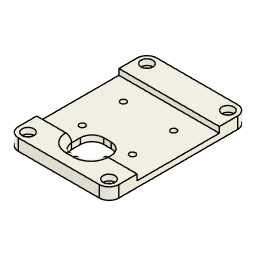
LINK-SHELF-to-B_ADPTOR (Autodesk Fusion 360 design; units mm, degrees)
Autodesk Fusion 360 part; units mm, degrees
sketch "Sketch1" plane through (0, 0, 9.3444) normal (0, 0, 1) x (1, 0, 0)
  circle A0 centre (-20.83, 96.1191) radius 1.5
  circle A1 centre (-20.83, 157.2691) radius 1.5
  circle A2 centre (20.83, 96.1191) radius 1.5
  circle A3 centre (20.83, 157.2691) radius 1.5
  line L0 (-15, 155.8968) -> (-15, 157.1191)
  line L1 (-15, 157.1191) -> (15, 157.1191)
  line L2 (15, 157.1191) -> (15, 155.8968)
  line L3 (15, 155.8968) -> (-15, 155.8968)
  arc A4 (25.83, 157.2691) -> (20.83, 162.2691) centre (20.83, 157.2691) ccw
  line L4 (20.83, 162.2691) -> (-20.83, 162.2691)
  arc A5 (-20.83, 162.2691) -> (-25.83, 157.2691) centre (-20.83, 157.2691) ccw
  line L5 (-25.83, 157.2691) -> (-25.83, 96.1191)
  arc A6 (-25.83, 96.1191) -> (-20.83, 91.1191) centre (-20.83, 96.1191) ccw
  line L6 (-20.83, 91.1191) -> (20.83, 91.1191)
  arc A7 (20.83, 91.1191) -> (25.83, 96.1191) centre (20.83, 96.1191) ccw
  line L7 (25.83, 96.1191) -> (25.83, 157.2691)
  line L8 (11.75, 110.7057) -> (11.75, 99.7057)
  line L9 (11.75, 99.7057) -> (0.75, 99.7057)
  line L10 (0.75, 99.7057) -> (0.75, 110.7057)
  line L11 (-0.75, 110.7057) -> (-0.75, 99.7057)
  line L12 (-0.75, 99.7057) -> (-11.75, 99.7057)
  line L13 (-11.75, 99.7057) -> (-11.75, 110.7057)
  line L14 (8.8, 110.7057) -> (11.75, 110.7057)
  line L15 (0.75, 110.7057) -> (3.7, 110.7057)
  line L16 (-3.7, 110.7057) -> (-0.75, 110.7057)
  line L17 (-11.75, 110.7057) -> (-8.8, 110.7057)
  line L18 (3.7, 110.7057) -> (3.7, 139.7691)
  line L19 (3.7, 139.7691) -> (8.8, 139.7691)
  line L20 (8.8, 139.7691) -> (8.8, 110.7057)
  line L21 (-8.8, 110.7057) -> (-8.8, 139.7691)
  line L22 (-8.8, 139.7691) -> (-3.7, 139.7691)
  line L23 (-3.7, 139.7691) -> (-3.7, 110.7057)
extrude "Extrude1" add sketch "Sketch1" along normal blind 3 contours L0 L1 L2 L3 | A4 L4 A5 L5 A6 L6 A7 L7 | L8 L9 L10 L14 L15 L18 L19 L20 | L11 L12 L13 L16 L17 L21 L22 L23
sketch "Sketch2" plane through (0, 0, 12.3444) normal (0, 0, 1) x (-1, 0, 0)
  circle A0 centre (20.83, -157.2691) radius 1.5
  circle A1 centre (20.83, -96.1191) radius 1.5
  circle A2 centre (-20.83, -157.2691) radius 1.5
  circle A3 centre (-20.83, -96.1191) radius 1.5
  line L0 (-25.83, -96.1191) -> (-25.83, -157.2691)
  arc A4 (-25.83, -157.2691) -> (-20.83, -162.2691) centre (-20.83, -157.2691) ccw
  line L1 (-20.83, -162.2691) -> (20.83, -162.2691)
  arc A5 (20.83, -162.2691) -> (25.83, -157.2691) centre (20.83, -157.2691) ccw
  line L2 (25.83, -157.2691) -> (25.83, -96.1191)
  arc A6 (25.83, -96.1191) -> (20.83, -91.1191) centre (20.83, -96.1191) ccw
  line L3 (20.83, -91.1191) -> (-20.83, -91.1191)
  arc A7 (-20.83, -91.1191) -> (-25.83, -96.1191) centre (-20.83, -96.1191) ccw
  line L4 (-25.83, -126.6941) -> (25.83, -126.6941) construction
  line L5 (0, -126.6941) -> (0, -105.5441) construction
  line L6 (0, -126.6941) -> (0, -147.8441) construction
  line L7 (-25.83, -105.5441) -> (25.83, -105.5441)
  line L8 (25.83, -105.5441) -> (25.83, -147.8441)
  line L9 (25.83, -147.8441) -> (-25.83, -147.8441)
  line L10 (-25.83, -147.8441) -> (-25.83, -105.5441)
  dimension "d41" = 21.15
  dimension "d42" = 21.15
  constraint midpoint L0 L4.start
  constraint midpoint L2 L4.end
  constraint midpoint L4 L5.start
  constraint perpendicular L4 L5
  constraint perpendicular L4 L6
  constraint horizontal L7
  constraint vertical L8
  constraint horizontal L9
  constraint vertical L10
  constraint coincident L2 L8.end
  constraint coincident L0 L7.start
  measures "d41" distance of L5.start L5.end
  measures "d42" distance of L5.start L6.end
extrude "Extrude2" add sketch "Sketch2" along normal blind 3 contours L0 L2 A6 L3 A7 L7 | L0 A4 L1 A5 L2 L9
sketch "Sketch3" plane through (0, 0, 15.3444) normal (0, 0, 1) x (-1, 0, 0)
  circle A0 centre (-20.83, -157.2691) radius 1.5
  circle A1 centre (20.83, -157.2691) radius 1.5
  line L0 (25.83, -147.8441) -> (-25.83, -147.8441)
  line L1 (-25.83, -147.8441) -> (-25.83, -157.2691)
  arc A2 (-25.83, -157.2691) -> (-20.83, -162.2691) centre (-20.83, -157.2691) ccw
  line L2 (-20.83, -162.2691) -> (20.83, -162.2691)
  arc A3 (20.83, -162.2691) -> (25.83, -157.2691) centre (20.83, -157.2691) ccw
  line L3 (25.83, -157.2691) -> (25.83, -147.8441)
  circle A4 centre (-20.83, -96.1191) radius 1.5
  circle A5 centre (20.83, -96.1191) radius 1.5
  line L4 (-25.83, -105.5441) -> (25.83, -105.5441)
  line L5 (25.83, -105.5441) -> (25.83, -96.1191)
  arc A6 (25.83, -96.1191) -> (20.83, -91.1191) centre (20.83, -96.1191) ccw
  line L6 (20.83, -91.1191) -> (-20.83, -91.1191)
  arc A7 (-20.83, -91.1191) -> (-25.83, -96.1191) centre (-20.83, -96.1191) ccw
  line L7 (-25.83, -96.1191) -> (-25.83, -105.5441)
  circle A8 centre (-20.83, -157.2691) radius 3.05
  circle A9 centre (20.83, -157.2691) radius 3.05
  circle A10 centre (-20.83, -96.1191) radius 3.05
  circle A11 centre (20.83, -96.1191) radius 3.05
  dimension "d45" = 6.1
  dimension "d46" = 6.1
  dimension "d47" = 6.1
  dimension "d48" = 6.1
  constraint concentric A0 A8
  constraint concentric A1 A9
  constraint concentric A4 A10
  constraint concentric A5 A11
  measures "d45" diameter of A8
  measures "d46" diameter of A9
  measures "d47" diameter of A10
  measures "d48" diameter of A11
extrude "Extrude3" cut sketch "Sketch3" against normal blind 3 contours A8 | A9 | A10 | A11
sketch "Sketch4" plane through (0, 0, 12.3444) normal (0, 0, 1) x (-1, 0, 0)
  line L0 (-25.83, -147.8441) -> (25.83, -147.8441)
  line L1 (25.83, -147.8441) -> (25.83, -105.5441)
  line L2 (25.83, -105.5441) -> (-25.83, -105.5441)
  line L3 (-25.83, -105.5441) -> (-25.83, -147.8441)
  line L4 (-25.83, -126.6941) -> (25.83, -126.6941) construction
  line L5 (0, -105.5441) -> (0, -147.8441) construction
  line L6 (0, -126.6941) -> (-25.83, -105.5441) construction
  line L7 (0, -126.6941) -> (25.83, -105.5441) construction
  circle A0 centre (-12.915, -116.1191) radius 1.5
  circle A1 centre (12.915, -116.1191) radius 1.5
  circle A2 centre (-12.915, -137.2691) radius 1.5
  circle A3 centre (12.915, -137.2691) radius 1.5
  dimension "d51" = 3
  dimension "d52" = 3
  constraint midpoint L3 L4.start
  constraint midpoint L1 L4.end
  constraint midpoint L2 L5.start
  constraint midpoint L0 L5.end
  constraint midpoint L5 L6.start
  constraint coincident L2.end L3.start
  constraint coincident L1.end L2.start
  constraint midpoint L6 A0.centre
  constraint midpoint L7 A1.centre
  constraint symmetric L4 A0 A2
  constraint symmetric L4 A1 A3
  measures "d51" diameter of A0
  measures "d52" diameter of A1
extrude "Extrude4" cut sketch "Sketch4" against normal blind 3 contours A0 | A1 | A2 | A3
sketch "Sketch5" plane through (0, 0, 12.3444) normal (0, 0, 1) x (-1, 0, 0)
  circle A0 centre (-12.915, -116.1191) radius 1.5
  circle A1 centre (12.915, -116.1191) radius 1.5
  circle A2 centre (-12.915, -137.2691) radius 1.5
  circle A3 centre (12.915, -137.2691) radius 1.5
  line L0 (-25.83, -147.8441) -> (25.83, -147.8441)
  line L1 (25.83, -147.8441) -> (25.83, -105.5441)
  line L2 (25.83, -105.5441) -> (-25.83, -105.5441)
  line L3 (-25.83, -105.5441) -> (-25.83, -147.8441)
  line L4 (0, -105.5441) -> (0, -120) construction
  line L5 (-12.915, -116.1191) -> (-7.915, -116.1191) construction
  line L6 (12.915, -116.1191) -> (7.915, -116.1191) construction
  line L7 (-7.915, -110.1191) -> (-7.915, -105.5441)
  line L8 (7.915, -110.1191) -> (7.915, -105.5441)
  line L9 (1.915, -116.1191) -> (-1.915, -116.1191)
  arc A4 (-7.915, -110.1191) -> (-1.915, -116.1191) centre (-1.915, -110.1191) ccw
  arc A5 (1.915, -116.1191) -> (7.915, -110.1191) centre (1.915, -110.1191) ccw
  dimension "d55" = 5
  dimension "d56" = 5
  dimension "d57" = 6
  constraint midpoint L2 L4.start
  constraint perpendicular L2 L4
  constraint coincident A0.centre L5.start
  constraint perpendicular L4 L5
  constraint coincident A1.centre L6.start
  constraint horizontal L6
  constraint coincident L2 L7.end
  constraint perpendicular L2 L7
  constraint coincident L2 L8.end
  constraint perpendicular L2 L8
  constraint coincident L5.end L7
  constraint coincident L5.end L9
  constraint tangent L7 A4
  constraint tangent L9 A4
  constraint coincident L6.end L9
  constraint coincident L6.end L8
  constraint tangent L9 A5
  constraint tangent L8 A5
  constraint equal A4 A5
  measures "d55" distance of A0.centre L5.end
  measures "d56" distance of A1.centre L6.end
  measures "d57" radius of A4
extrude "Extrude5" cut sketch "Sketch5" against normal blind 3 contours L2 L7 L8 L9 A4 A5
sketch "Sketch6" plane through (0, 0, 15.3444) normal (0, 0, 1) x (-1, 0, 0)
  circle A0 centre (-20.83, -96.1191) radius 3.05
  circle A1 centre (20.83, -96.1191) radius 3.05
  line L0 (-25.83, -105.5441) -> (25.83, -105.5441)
  line L1 (25.83, -105.5441) -> (25.83, -96.1191)
  arc A2 (25.83, -96.1191) -> (20.83, -91.1191) centre (20.83, -96.1191) ccw
  line L2 (20.83, -91.1191) -> (-20.83, -91.1191)
  arc A3 (-20.83, -91.1191) -> (-25.83, -96.1191) centre (-20.83, -96.1191) ccw
  line L3 (-25.83, -96.1191) -> (-25.83, -105.5441)
  line L4 (-7.915, -110.1191) -> (-7.915, -105.5441)
  line L5 (-7.915, -105.5441) -> (-25.83, -105.5441)
  line L6 (-25.83, -105.5441) -> (-25.83, -147.8441)
  line L7 (-25.83, -147.8441) -> (25.83, -147.8441)
  line L8 (25.83, -147.8441) -> (25.83, -105.5441)
  line L9 (25.83, -105.5441) -> (7.915, -105.5441)
  line L10 (7.915, -105.5441) -> (7.915, -110.1191)
  arc A4 (1.915, -116.1191) -> (7.915, -110.1191) centre (1.915, -110.1191) ccw
  line L11 (1.915, -116.1191) -> (-1.915, -116.1191)
  arc A5 (-7.915, -110.1191) -> (-1.915, -116.1191) centre (-1.915, -110.1191) ccw
  circle A6 centre (-12.915, -116.1191) radius 1.5
  circle A7 centre (12.915, -116.1191) radius 1.5
  circle A8 centre (-12.915, -137.2691) radius 1.5
  circle A9 centre (12.915, -137.2691) radius 1.5
  line L12 (7.915, -116.1191) -> (-7.915, -116.1191)
  line L13 (-7.915, -116.1191) -> (-7.915, -105.7061)
  line L14 (-1.915, -99.7061) -> (1.915, -99.7061)
  line L15 (7.915, -105.7061) -> (7.915, -116.1191)
  arc A10 (7.915, -105.7061) -> (1.915, -99.7061) centre (1.915, -105.7061) ccw
  arc A11 (-1.915, -99.7061) -> (-7.915, -105.7061) centre (-1.915, -105.7061) ccw
  point P0 (7.915, -99.7061)
  dimension "d332" = 16.413
  dimension "d333" = 6
  constraint horizontal L12
  constraint vertical L13
  constraint horizontal L14
  constraint vertical L15
  constraint coincident P0 L14
  constraint coincident P0 L15
  constraint tangent L14 A10
  constraint tangent L15 A10
  constraint tangent L13 A11
  constraint tangent L14 A11
  constraint equal A10 A11
  measures "d332" distance of L12.start P0
  measures "d333" radius of A10
extrude "Extrude6" cut sketch "Sketch6" against normal blind 6 contours L0 L14 A10 A11
fillet "Fillet1" radius 3 3 edges at (6.1, 101.4065, 15.3444) (0, 99.7061, 15.3444) (-6.1, 101.4065, 15.3444)
equation "d332 = ( ( 10.575 * 2 ) * 1 mm ) - 4.737 mm"
